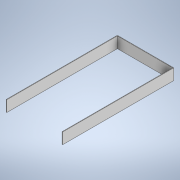
# Autodesk Inventor part: vibro_bed_stl
Saved by Autodesk Inventor 2021 (Build 250183000, 183)
## iProperties
Created: 2020-07-13
Part Number: vibro_bed_stl
Material: Generic
Document SubType Name: Modeling
Designer: dwer2
Density: 1 g/cm^3
Appearance: Default
Author: dwer2
Autodesk Inventor part; units mm, degrees
ref_plane "YZ Plane" through (0, 0, 0) normal (1, 0, 0) x (0, 1, 0)
ref_plane "XZ Plane" through (0, 0, 0) normal (0, 1, 0) x (-1, 0, 0)
ref_plane "XY Plane" through (0, 0, 0) normal (0, 0, 1) x (1, 0, 0)
sketch "Sketch1" plane through (0, 0, 0) normal (0, 1, 0) x (-1, 0, 0)
  line L0 (102, 0) -> (0, 0)
  line L1 (0, 0) -> (0, 201)
  line L2 (0, 201) -> (1, 201)
  line L3 (1, 201) -> (1, 1)
  line L4 (1, 1) -> (101, 1)
  line L5 (101, 1) -> (101, 201)
  line L6 (101, 201) -> (102, 201)
  line L7 (102, 201) -> (102, 0)
  dimension "d0" = 1
  dimension "d1" = 1
  dimension "d2" = 100
  dimension "d3" = 102
  dimension "d4" = 1
  dimension "d5" = 201
  constraints: 16 end point, 5 perpendicular, 2 point on line, 1 horizontal
  measures "d0" distance of L1.end L2.end
  measures "d1" distance of L5.end L6.end
  measures "d2" distance of L3.end L4.end
  measures "d3" distance of L0.start L0.end
  measures "d4" distance between parallel lines of L0 L4
  measures "d5" distance of L0.end L1.end
extrude "Extrusion1" add sketch "Sketch1" along normal blind 20
body "Solid1"
